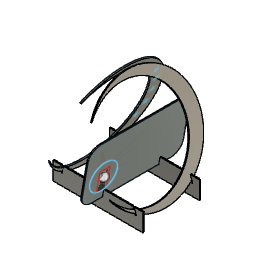
レーザー２ v4 (Autodesk Fusion 360 design; units mm, degrees)
Autodesk Fusion 360 part; units mm, degrees
sketch "スケッチ1" plane through (0, 0, 0) normal (0, 0, 1) x (1, 0, 0)
  arc A0 (90, 100) -> (150.8761, -16.1766) centre (31.7692, -4.5504) ccw
  arc A1 (90, 100) -> (150.8761, -16.1766) centre (46.8979, 3.377) ccw
extrude "押し出し1" add sketch "スケッチ1" along normal blind 2.45 makes body 1
sketch "スケッチ2" plane through (0, 0, 0) normal (1, 0, 0) x (0, 1, 0)
sketch "スケッチ3" plane through (0, 0, 0) normal (0, 1, 0) x (1, 0, 0)
  line L0 (-300, 0) -> (-180, 0)
  line L1 (-300, -20) -> (-300, 0)
  line L2 (-180, 0) -> (-180, -20)
  line L3 (-290, -20) -> (-293.4202, -10.6031)
  line L4 (-290, -20) -> (-280, -20) construction
  line L5 (-293.4202, -10.6031) -> (-291.118, -9.7651)
  line L6 (-291.118, -9.7651) -> (-287.3928, -20)
  line L7 (-290, -20) -> (-300, -20)
  line L8 (-190, -20) -> (-186.5798, -10.6031)
  line L9 (-190, -20) -> (-180, -20) construction
  line L10 (-186.5798, -10.6031) -> (-188.882, -9.7651)
  line L11 (-188.882, -9.7651) -> (-192.6072, -20)
  line L12 (-180, -20) -> (-190, -20)
  line L13 (-192.6072, -20) -> (-287.3928, -20)
  dimension "d4" = 110
  dimension "d5" = 10
  dimension "d7" = 2.45
  dimension "d8" = 70
  dimension "d9" = 10
  dimension "d10" = 2.45
  constraint horizontal L0
  constraint perpendicular L0 L1
  constraint perpendicular L0 L2
  constraint perpendicular L1 L12
  constraint horizontal L4
  constraint coincident L3.start L12
  constraint perpendicular L3 L5
  constraint collinear L7 L12
  constraint horizontal L9
  constraint perpendicular L8 L10
  constraint perpendicular L10 L11
  constraint collinear L12 L13
  measures "d4" angle of L3 L4
  measures "d5" distance of L3.start L3.end
  measures "d7" distance of L3.end L5.end
  measures "d8" angle of L8 L9
  measures "d9" distance of L8.start L8.end
  measures "d10" distance of L8.end L10.end
extrude "押し出し2" add sketch "スケッチ3" along normal blind 2.45 separate body makes body 2
move_body "移動1" bodies 1 to x (0.209359, -0.739007, 0.640342) y (0.282585, -0.581188, -0.763129) z (0.936117, 0.340719, 0.087156) at (-172.238, -35.0051, 134.0301)
copy_body "ボディのコピーと貼り付け1" bodies 1 makes body 3
move_body "移動2" bodies 3 to x (1, 0, 0) y (0, 1, 0) z (0, 0, 1) at (0, 0, 0)
move_body "移動3" bodies 1 to x (0.849962, -0.328858, -0.411604) y (0.308059, 0.94401, -0.118089) z (0.427393, -0.026427, 0.90368) at (-159.7688, -28.4081, -94.2868)
move_body "移動4" bodies 3 to x (0.926447, 0.350468, 0.137359) y (-0.359548, 0.931929, 0.047258) z (-0.111446, -0.093169, 0.989393) at (-47.84, 159.5147, -4.0655)
move_body "移動5" bodies 3 to x (0.775281, -0.631237, 0.021875) y (0.610218, 0.757505, 0.231991) z (-0.163012, -0.16651, 0.972472) at (-3.0828, -98.4035, 2.6222)
delete_body "RemoveBody1" bodies 2
sketch "スケッチ4" plane through (0, 0, 0) normal (0, 1, 0) x (1, 0, 0)
  line L0 (-75, 0) -> (-325, 0)
  line L1 (-325, -50) -> (-325, 0)
  line L2 (-325, -30.1758) -> (-287.7338, -30.1758)
  line L3 (-287.7338, -30.1758) -> (-293.2061, -15.1408)
  line L4 (-75, 0) -> (-75, -30.1758)
  line L5 (-75, -30.1758) -> (-112.9323, -30.1758)
  line L6 (0, 0) -> (200, 0)
  line L7 (200, 0) -> (200, -40)
  line L8 (0, -40) -> (0, 0)
  line L9 (20, -40) -> (22.45, -40)
  line L10 (180, -40) -> (177.55, -40)
  line L11 (180, -40) -> (185.1303, -25.9046)
  line L12 (180, -40) -> (195, -40) construction
  line L13 (185.1303, -25.9046) -> (182.8281, -25.0667)
  line L14 (177.55, -40) -> (182.8281, -25.0667)
  line L15 (200, -40) -> (180, -40)
  line L16 (20, -40) -> (17.3953, -25.2279)
  line L17 (20, -40) -> (35, -40) construction
  line L18 (19.8081, -24.8024) -> (22.45, -40)
  line L19 (17.3953, -25.2279) -> (19.8091, -24.8083)
  line L20 (177.55, -40) -> (22.45, -40)
  line L21 (20, -40) -> (0, -40)
  dimension "d13" = 16
  dimension "d14" = 70
  dimension "d15" = 40
  dimension "d16" = 2.45
  dimension "d17" = 2.45
  dimension "d21" = 70
  dimension "d22" = 15
  dimension "d23" = 2.45
  dimension "d24" = 100
  dimension "d25" = 15
  dimension "d26" = 2.45
  dimension "d27" = 2.45
  constraint perpendicular L0 L1
  constraint coincident L1 L2.start
  constraint perpendicular L1 L2
  constraint perpendicular L0 L4
  constraint perpendicular L4 L5
  constraint coincident L6.start L8.end
  constraint horizontal L6
  constraint perpendicular L6 L7
  constraint perpendicular L7 L15
  constraint perpendicular L6 L8
  constraint coincident L9.start L15
  constraint parallel L9 L15
  constraint perpendicular L7 L10
  constraint horizontal L12
  constraint perpendicular L11 L13
  constraint collinear L15 L20
  constraint horizontal L17
  constraint perpendicular L18 L19
  constraint collinear L20 L21
  measures "d13" distance of L2.end L3.end
  measures "d14" angle of L2 L3
  measures "d15" distance of L6.end L7.end
  measures "d16" distance of L9.start L9.end
  measures "d17" distance of L10.start L10.end
  measures "d21" angle of L11 L12
  measures "d22" distance of L10.start L11.end
  measures "d23" distance of L11.end L13.end
  measures "d24" angle of L16 L17
  measures "d25" distance of L9.start L16.end
  measures "d26" distance of L16.end L18.start
  measures "d27" distance of L16.end L19.end
extrude "押し出し3" add sketch "スケッチ4" along normal blind 2.5 separate body contours L6 L7 L8 L11 L13 L14 L15 L16 L18 L19 L20 L21 makes body 4
extrude "押し出し4" add 1 faces at (-163.5316, 138.9474, 154.4827) along direction (0.921229, -0.01954, 0.38853) blind 0.5 on bodies 3 bodies 3
extrude "押し出し5" add 1 faces at (-246.5107, 78.3885, 133.2448) along direction (0.937875, 0.011489, -0.346784) blind 0.5 on bodies 1 bodies 1
copy_body "ボディのコピーと貼り付け2" bodies 4 makes body 5
move_body "移動6" bodies 5 to x (1, 0, 0) y (0, 1, 0) z (0, 0, 1) at (0, -125, 0)
move_body "移動7" bodies 3 to x (1, 0, 0) y (0, 1, 0) z (0, 0, 1) at (299.7727, -106.3809, -8.3339)
move_body "移動8" bodies 1 to x (0.996048, -0.009051, 0.088359) y (0.009328, 0.999953, -0.00272) z (-0.08833, 0.003533, 0.996085) at (308.1374, -37.0781, 38.55)
move_body "移動9" bodies 3 to x (0.999275, 0.020948, -0.031787) y (-0.021219, 0.999741, -0.008216) z (0.031606, 0.008885, 0.999461) at (-3.1778, 5.8224, 6.452)
move_body "移動10" bodies 1 to x (0.996043, 0.000658, -0.08887) y (-0.000726, 0.999999, -0.000733) z (0.08887, 0.000794, 0.996043) at (-16.5896, 3.0726, -10.1499)
move_body "移動11" bodies 1 to x (1, 0, 0) y (0, 1, 0) z (0, 0, 1) at (10.7667, -0.0061, 0.2779)
sketch "スケッチ5" plane through (0, 0, 0) normal (0, 1, 0) x (1, 0, 0)
  line L0 (110, -40) -> (107.3953, -25.2279)
  line L1 (110, -40) -> (125, -40) construction
  line L2 (107.3953, -25.2279) -> (109.8081, -24.8024)
  line L3 (109.8081, -24.8024) -> (112.4878, -40)
  line L4 (112.4878, -40) -> (110, -40)
  dimension "d34" = 100
  dimension "d35" = 15
  dimension "d36" = 2.45
  constraint horizontal L1
  constraint perpendicular L0 L2
  constraint perpendicular L2 L3
  constraint coincident L1 L3.end
  measures "d34" angle of L0 L1
  measures "d35" distance of L0.start L0.end
  measures "d36" distance of L0.end L2.end
extrude "押し出し6" cut sketch "スケッチ5" along normal blind 25 and the other way blind 170 bodies 4 5
sketch "スケッチ6" plane through (0, 0, 0) normal (1, 0, 0) x (0, 1, 0)
  line L0 (225, 0) -> (50, 0)
  line L1 (25, 25) -> (25, 100)
  line L2 (50, 125) -> (225, 125)
  line L3 (250, 100) -> (250, 25)
  arc A0 (250, 100) -> (225, 125) centre (225, 100) ccw
  arc A1 (225, 0) -> (250, 25) centre (225, 25) ccw
  arc A2 (25, 25) -> (50, 0) centre (50, 25) ccw
  arc A3 (50, 125) -> (25, 100) centre (50, 100) ccw
  dimension "d41" = 25
  constraint horizontal L0
  constraint vertical L1
  constraint horizontal L2
  constraint vertical L3
  constraint tangent L2 A0
  constraint tangent L3 A0
  constraint tangent L0 A1
  constraint tangent L3 A1
  constraint equal A0 A1
  constraint tangent L0 A2
  constraint tangent L1 A2
  constraint equal A0 A2
  constraint tangent L1 A3
  constraint tangent L2 A3
  constraint equal A0 A3
  measures "d41" radius of A0
extrude "押し出し7" add sketch "スケッチ6" along normal blind 2.5 separate body makes body 6
move_body "移動12" bodies 6 to x (0.984808, 0, -0.173648) y (0, 1, 0) z (0.173648, 0, 0.984808) at (107.8608, -200, 25.5494)
sketch "スケッチ7" plane through (5.7742, 0.0136, -2.1385) normal (-0.937751, -0.002201, 0.347302) x (0.002347, -0.999997, 0)
  arc A0 (147.7599, 218.7932) -> (172.303, 89.9501) centre (61.6953, 135.6398) ccw
  arc A1 (147.7599, 218.7932) -> (172.303, 89.9501) centre (78.4734, 138.8359) ccw
  dimension "d44" = 15
sketch "スケッチ8" plane through (102.7012, 0, -18.109) normal (0.984808, 0, -0.173648) x (0, 1, 0)
  arc A0 (50, 143.891) -> (25, 168.891) centre (25, 143.891) ccw
  line L0 (25, 168.891) -> (-150, 168.891)
  arc A1 (-150, 168.891) -> (-175, 143.891) centre (-150, 143.891) ccw
  line L1 (-175, 143.891) -> (-175, 68.891)
  arc A2 (-175, 68.891) -> (-150, 43.891) centre (-150, 68.891) ccw
  line L2 (-150, 43.891) -> (25, 43.891)
  arc A3 (25, 43.891) -> (50, 68.891) centre (25, 68.891) ccw
  line L3 (50, 68.891) -> (50, 143.891)
  circle A4 centre (-131.596, 90.7547) radius 30.5151
